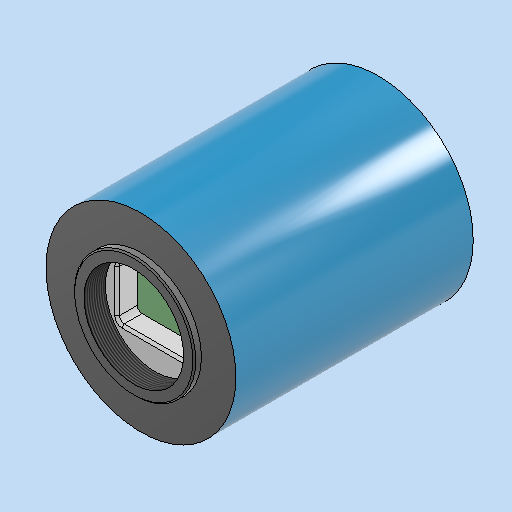
# Autodesk Inventor part: RisingCam-IMX571
Saved by Autodesk Inventor 2025 (Build 290162000, 162)
## iProperties
Created: 2025-02-20
Part Number: RisingCam-IMX571
Material: Generic
Document SubType Name: Modeling
Designer: kuzmin
Density: 1 g/cm^3
Appearance: Default
Author: kuzmin
Autodesk Inventor part; units mm, degrees
ref_plane "YZ Plane" through (0, 0, 0) normal (1, 0, 0) x (0, 1, 0)
ref_plane "XZ Plane" through (0, 0, 0) normal (0, 1, 0) x (-1, 0, 0)
ref_plane "XY Plane" through (0, 0, 0) normal (0, 0, 1) x (1, 0, 0)
sketch "Sketch1" plane through (0, 0, 0) normal (0, 0, 1) x (1, 0, 0)
  circle A0 centre (0, 0) radius 40
  dimension "d0" = 80
  constraints: 1 centre point, 1 coincident
  measures "d0" diameter of A0
extrude "Extrusion1" add sketch "Sketch1" along normal blind 100
sketch "Sketch2" plane through (0, 0, 100) normal (0, 0, 1) x (1, 0, 0)
  circle A0 centre (0, 0) radius 25.5
  dimension "d3" = 51
  constraints: 1 centre point, 1 coincident
  measures "d3" diameter of A0
extrude "Extrusion2" add sketch "Sketch2" along normal blind 3
chamfer "Chamfer1" distance 0.6 angle 45 1 edges at (-25.5, 0, 103)
sketch "Sketch3" plane through (0, 0, 103) normal (0, 0, 1) x (1, 0, 0)
  circle A0 centre (0, 0) radius 21
  dimension "d9" = 42
  constraints: 1 centre point, 1 coincident
  measures "d9" diameter of A0
extrude "SensorCutout" cut sketch "Sketch3" against normal blind 17.5
thread "Thread1" size "M42x1" class "6H" standard "ANSI Metric M Profile" full length
sketch "Sketch4" plane through (0, 0, 85.5) normal (0, 0, 1) x (1, 0, 0)
  line L0 (-16, 11) -> (16, 11)
  line L1 (16, 11) -> (16, -11)
  line L2 (16, -11) -> (-16, -11)
  line L3 (-16, -11) -> (-16, 11)
  circle A0 centre (0, 0) radius 21 projected
  point P0 (16, 0)
  point P1 (0, 11)
  dimension "d14" = 32
  dimension "d15" = 22
  constraints: 8 end point, 2 midpoint, 2 parallel, 1 horizontal, 1 horizontal alignment, 1 perpendicular, 1 vertical alignment
  measures "d14" distance of L0.start L0.end
  measures "d15" distance of L0.end L1.end
extrude "SensorFrame" add sketch "Sketch4" along normal blind 8.5
fillet "Fillet1" radius 2 4 edges at (-16, 11, 89.75) (-16, -11, 89.75) (16, 11, 89.75) (16, -11, 89.75)
chamfer "Chamfer2" distance 1 angle 45 4 edges at (0, 11, 94) (16, 0, 94) (0, -11, 94) (-16, 0, 94)
body "Solid1"
